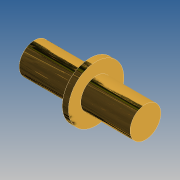
# Autodesk Inventor part: P002
Saved by Autodesk Inventor 2017 (Build 210142000, 142)
## iProperties
Created: 2018-10-19
Part Number: P002
Material: Bronze
Document SubType Name: Modeling
Designer: Gilles Mottiez
Density: 8.95 g/cm^3
Appearance: Laiton - Satiné
Description: Axe plateforme
Author: Gilles Mottiez
Autodesk Inventor part; units mm, degrees
ref_plane "YZ Plane" through (0, 0, 0) normal (1, 0, 0) x (0, 1, 0)
ref_plane "XZ Plane" through (0, 0, 0) normal (0, 1, 0) x (-1, 0, 0)
ref_plane "XY Plane" through (0, 0, 0) normal (0, 0, 1) x (1, 0, 0)
sketch "Sketch1" plane through (0, 0, 0) normal (0, 0, 1) x (1, 0, 0)
  line L0 (0, 0) -> (18, 0)
  line L1 (0, 0) -> (0, 2.5)
  line L2 (0, 2.5) -> (9, 2.5)
  line L3 (9, 2.5) -> (9, 4.5)
  line L4 (9, 4.5) -> (10, 4.5)
  line L5 (10, 4.5) -> (10, 2.5)
  line L6 (10, 2.5) -> (18, 2.5)
  line L7 (18, 2.5) -> (18, 0)
  dimension "d0" = 18
  dimension "d1" = 5
  dimension "d2" = 9
  dimension "d3" = 9
  dimension "d4" = 1
  constraints: 16 end point, 5 perpendicular, 2 point on line, 1 horizontal, 1 vertical
  measures "d0" distance of L0.start L0.end
  measures "d1" diameter of L2 L0
  measures "d2" diameter of L4 L0
  measures "d3" distance of L1.end L2.end
  measures "d4" distance of L3.end L4.end
revolve "Révolution1" add sketch "Sketch1" angle 360 about axis through (0, 0, 0) along (1, 0, 0)
